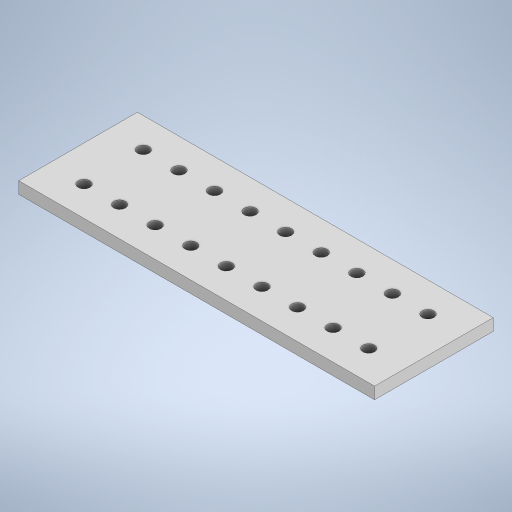
# Autodesk Inventor part: Lochplatte
Saved by Autodesk Inventor 2024 (Build 280153000, 153)
## iProperties
Created: 2023-08-23
Part Number: Lochplatte
Material: Generisch
Document SubType Name: Modeling
Designer: rapp
Density: 1 g/cm^3
Appearance: Vorgabe
Author: rapp
Autodesk Inventor part; units mm, degrees
ref_plane "YZ Plane" through (0, 0, 0) normal (1, 0, 0) x (0, 1, 0)
ref_plane "XZ Plane" through (0, 0, 0) normal (0, 1, 0) x (-1, 0, 0)
ref_plane "XY Plane" through (0, 0, 0) normal (0, 0, 1) x (1, 0, 0)
sketch "Skizze1" plane through (0, 0, 0) normal (0, 0, 1) x (1, 0, 0)
  line L0 (-150, -50) -> (150, -50)
  line L1 (150, -50) -> (150, 50)
  line L2 (150, 50) -> (-150, 50)
  line L3 (-150, 50) -> (-150, -50)
  line L4 (-210, 0) -> (210, 0) projected
  line L5 (0, -70) -> (0, 70) projected
  point P0 (0, 0)
  dimension "d0" = 300
  dimension "d1" = 100
  constraints: 8 end point, 2 parallel, 1 horizontal, 1 perpendicular, 2 other
  measures "d0" distance of L0.start L0.end
  measures "d1" distance of L2.end L0.start
extrude "Extrusion1" add sketch "Skizze1" along normal blind 10
sketch "Skizze2" plane through (0, 0, 10) normal (0, 0, 1) x (1, 0, 0)
  line L0 (-210, 0) -> (210, 0) projected
  line L1 (0, -70) -> (0, 70) projected
  line L2 (-150, 50) -> (-150, -50) projected
  point P0 (0, 0)
  point P1 (-120, -25)
  dimension "d4" = 25
  dimension "d5" = 30
  measures "d4" distance from line of point (-120, -25) L0
  measures "d5" distance from line of point (-120, -25) L2
hole "Bohrung1" at (-120, -25, 10) direction (0, 0, -1) diameter 10 end through all
pattern_linear "Rechteckige Anordnung1" count 9 spacing 30 along (1, 0, 0) count 2 spacing 50 along (0, 1, 0) of "Bohrung1"
